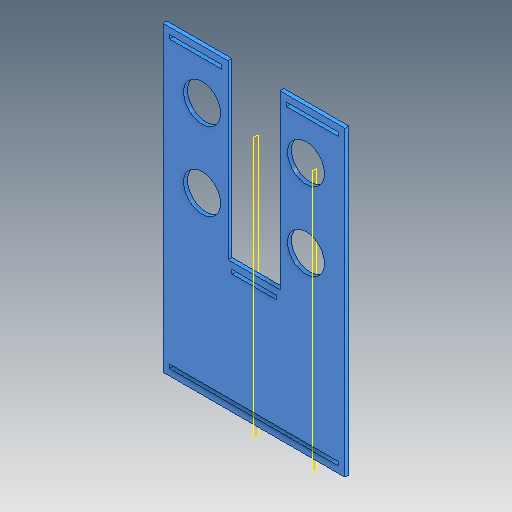
# Autodesk Inventor part: Ushape_bottom
Saved by Autodesk Inventor 2020 (Build 240168000, 168)
## iProperties
Created: 2021-05-10
Part Number: Ushape_bottom
Material: Generic
Document SubType Name: Modeling
Designer: Hsu Daniel
Density: 1 g/cm^3
Appearance: Cyan
Author: Hsu Daniel
Autodesk Inventor part; units mm, degrees
ref_plane "YZ Plane" through (0, 0, 0) normal (1, 0, 0) x (0, 1, 0)
ref_plane "XZ Plane" through (0, 0, 0) normal (0, 1, 0) x (-1, 0, 0)
ref_plane "XY Plane" through (0, 0, 0) normal (0, 0, 1) x (1, 0, 0)
sketch "Sketch1" plane through (0, 0, 0) normal (0, 0, 1) x (1, 0, 0)
  line L0 (0, 0) -> (140, 0)
  line L1 (140, 0) -> (140, 232.6)
  line L2 (140, 232.6) -> (90, 232.6)
  line L3 (90, 232.6) -> (90, 100)
  line L4 (90, 100) -> (50, 100)
  line L5 (50, 100) -> (50, 232.6)
  line L6 (50, 232.6) -> (0, 232.6)
  line L7 (0, 232.6) -> (0, 0)
  line L8 (30, 232.6) -> (30, 0) construction
  line L9 (70, 100) -> (70, 0) construction
  circle A0 centre (30, 192.6) radius 14 construction
  circle A1 centre (30, 152.6) radius 14 construction
  dimension "d3" = 40
  dimension "d6" = 28
  dimension "d7" = 40
  dimension "d8" = 40
  dimension "d9" = 132.6
  dimension "d10" = 100
  dimension "d36" = 20
  dimension "d37" = 50
  constraints: 20 end point, 6 perpendicular, 5 point on line, 2 centre point, 2 midpoint, 1 collinear, 1 equal radius, 1 horizontal, 1 vertical
  measures "d3" distance between parallel lines of L9 L8
  measures "d6" diameter of A0
  measures "d7" distance of A1.centre A0.centre
  measures "d8" distance from line of L6 A0.centre
  measures "d9" distance of L4.end L5.end
  measures "d10" distance of L9.start L9.end
  measures "d36" distance between parallel lines of L5 L8
  measures "d37" distance between parallel lines of L7 L5
extrude "Extrusion1" add sketch "Sketch1" along normal blind 3
ref_plane "Work Plane1" through (115, 0, 0) normal (1, 0, 0) x (0, 0, -1)
sketch "Sketch2" plane through (0, 0, 3) normal (0, 0, 1) x (1, 0, 0)
  line L0 (50, 232.6) -> (0, 232.6) construction
  line L1 (30, 232.6) -> (30, 50) construction
  line L2 (90, 100) -> (50, 100) construction
  line L3 (70, 100) -> (70, 0) construction
  line L4 (0, 0) -> (140, 0) construction
  circle A0 centre (30, 194.6) radius 14.25
  circle A1 centre (30, 134.6) radius 14.25
  circle A2 centre (30, 202.6) radius 4.6 construction
  circle A3 centre (110, 194.6) radius 14.25
  circle A4 centre (110, 134.6) radius 14.25
  line L5 (50, 100) -> (50, 232.6) projected
  dimension "d13" = 28.5
  dimension "d14" = 9.2
  dimension "d15" = 8
  dimension "d16" = 60
  dimension "d33" = 30
  dimension "d38" = 20
  constraints: 5 centre point, 4 end point, 3 point on line, 2 symmetric about line, 1 equal radius, 1 midpoint, 1 vertical, 4 other
  measures "d13" diameter of A0
  measures "d14" diameter of A2
  measures "d15" distance of A0.centre A2.centre
  measures "d16" distance of A1.centre A0.centre
  measures "d33" distance from line of L0 A2.centre
  measures "d38" distance between parallel lines of L5 L1
extrude "Extrusion2" cut sketch "Sketch2" against normal blind 10
sketch "Sketch3" plane through (0, 0, 3) normal (0, 0, 1) x (1, 0, 0)
  line L0 (5, 227.6) -> (45, 227.6)
  line L1 (45, 227.6) -> (45, 224.6)
  line L2 (45, 224.6) -> (5, 224.6)
  line L3 (5, 224.6) -> (5, 227.6)
  line L4 (53, 95) -> (87, 95)
  line L5 (87, 95) -> (87, 92)
  line L6 (87, 92) -> (53, 92)
  line L7 (53, 92) -> (53, 95)
  line L8 (5, 8) -> (135, 8)
  line L9 (135, 8) -> (135, 5)
  line L10 (135, 5) -> (5, 5)
  line L11 (5, 5) -> (5, 8)
  circle A0 centre (110, 194.6) radius 14.25 projected
  circle A1 centre (30, 134.6) radius 14.25 projected
  circle A2 centre (110, 134.6) radius 14.25 projected
  circle A3 centre (30, 194.6) radius 14.25 projected
  line L12 (50, 100) -> (50, 232.6) projected
  line L13 (50, 232.6) -> (0, 232.6) projected
  line L14 (0, 232.6) -> (0, 0) projected
  line L15 (0, 0) -> (140, 0) projected
  line L16 (140, 0) -> (140, 232.6) projected
  line L17 (140, 232.6) -> (90, 232.6) projected
  line L18 (90, 232.6) -> (90, 100) projected
  line L19 (90, 100) -> (50, 100) projected
  line L20 (90, 100) -> (50, 100) construction
  line L21 (70, 100) -> (70, 0) construction
  line L22 (0, 0) -> (140, 0) construction
  line L23 (135, 227.6) -> (95, 227.6)
  line L24 (95, 227.6) -> (95, 224.6)
  line L25 (95, 224.6) -> (135, 224.6)
  line L26 (135, 224.6) -> (135, 227.6)
  dimension "d20" = 5
  dimension "d21" = 5
  dimension "d22" = 5
  dimension "d23" = 3
  dimension "d24" = 5
  dimension "d25" = 3
  dimension "d26" = 3
  dimension "d27" = 3
  dimension "d28" = 5
  dimension "d29" = 3
  dimension "d30" = 5
  constraints: 34 end point, 6 parallel, 4 symmetric about line, 3 horizontal, 3 perpendicular, 2 midpoint, 1 point on line
  measures "d20" distance between parallel lines of L15 L10
  measures "d21" distance between parallel lines of L14 L11
  measures "d22" distance between parallel lines of L16 L9
  measures "d23" distance of L8.end L9.end
  measures "d24" distance between parallel lines of L19 L4
  measures "d25" distance of L4.end L5.end
  measures "d26" distance between parallel lines of L18 L5
  measures "d27" distance between parallel lines of L12 L7
  measures "d28" distance between parallel lines of L13 L0
  measures "d29" distance of L0.end L1.end
  measures "d30" distance between parallel lines of L12 L1
extrude "Extrusion3" cut sketch "Sketch3" against normal blind 10 contours L0 L1 L2 L3 | L4 L5 L6 L7 | L8 L9 L10 L11 | L26 L25 L24 L23
ref_plane "Work Plane2" through (70, 0, 0) normal (1, 0, 0) x (0, 0, -1)
equation "\"d3\" = 0.5 * marshdistance"
equation "\"d9\" = sidewallL"
equation "\"d10\" = Uthick"
equation "\"d36\" = 0.5 * Utip"
equation "\"d16\" = marshmarshD"
equation "\"d33\" = marshedgeD"
equation "\"d38\" = 0.5 * Utip"
equation "\"thick\" = 0.5"
equation "\"lrlr\" = 19"
equation "\"lrmid\" = 19.9"
equation "\"lrdepth\" = 3.3"
equation "\"mlr\" = 16.6"
equation "\"mmid\" = 24.7"
equation "\"mdepth\" = 4.5"
equation "\"lrltotal\" = 126.6"
equation "\"mltotal\" = 126.6"
equation "\"lrbetween\" = 52.1"
equation "\"mbetween\" = 49.5"
equation "\"toler\" = 1"
equation "\"tight\" = 0.08"
equation "\"stuckw\" = 6"
equation "\"sidewallL\" = 132.6"
equation "\"heaterH\" = 117.3"
equation "\"Uthick\" = 100"
equation "\"marshmarshD\" = 60"
equation "\"marshedgeD\" = 30"
equation "\"stickL\" = 3.5"
equation "\"wireH\" = 25"
equation "\"marshdistance\" = 80"
equation "\"Utip\" = 40"
body "Solid1"
